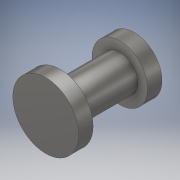
# Autodesk Inventor part: Rivet
Saved by Autodesk Inventor 2018 (Build 220112000, 112)
## iProperties
Created: 2018-02-27
Part Number: Rivet
Material: Stainless Steel
Document SubType Name: Modeling
Designer: 232963
Density: 8 g/cm^3
Appearance: Semi-Polished
Author: 232963
Autodesk Inventor part; units mm, degrees
ref_plane "YZ Plane" through (0, 0, 0) normal (1, 0, 0) x (0, 1, 0)
ref_plane "XZ Plane" through (0, 0, 0) normal (0, 1, 0) x (-1, 0, 0)
ref_plane "XY Plane" through (0, 0, 0) normal (0, 0, 1) x (1, 0, 0)
sketch "Sketch1" plane through (0, 0, 0) normal (0, 0, 1) x (1, 0, 0)
  circle A0 centre (0, 0) radius 2.2225
  dimension "d0" = 4.445
  constraints: 1 centre point, 1 coincident
  measures "d0" diameter of A0
extrude "Extrusion1" add sketch "Sketch1" along normal mid plane 7.366
sketch "Sketch2" plane through (0, 0, 3.683) normal (0, 0, 1) x (1, 0, 0)
  circle A0 centre (0, 0) radius 2.2225 projected
  circle A1 centre (0, 0) radius 4.064
  dimension "d3" = 8.128
  constraints: 1 centre point, 1 coincident
  measures "d3" diameter of A1
extrude "Extrusion2" add sketch "Sketch2" along normal blind 1.778 contours A0 | A1
sketch "Sketch3" plane through (0, 0, -3.683) normal (0, 0, -1) x (-1, 0, 0)
  circle A0 centre (0, 0) radius 3.429
  dimension "d6" = 6.858
  constraints: 1 centre point, 1 coincident
  measures "d6" diameter of A0
extrude "Extrusion3" add sketch "Sketch3" along normal blind 1.778
body "Solid1"
